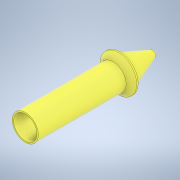
# Autodesk Inventor part: Static Marker Barrel
Saved by Autodesk Inventor 2022.2 (Build 262287010, 287A)
## iProperties
Created: 2022-02-09
Part Number: Static Marker Barrel
Material: ABS Plastic
Document SubType Name: Modeling
Designer: smiku
Density: 1.06 g/cm^3
Appearance: Smooth - Yellow
Author: smiku
Autodesk Inventor part; units mm, degrees
ref_plane "YZ Plane" through (0, 0, 0) normal (1, 0, 0) x (0, 1, 0)
ref_plane "XZ Plane" through (0, 0, 0) normal (0, 1, 0) x (-1, 0, 0)
ref_plane "XY Plane" through (0, 0, 0) normal (0, 0, 1) x (1, 0, 0)
sketch "Sketch1" plane through (0, 0, 0) normal (0, 0, 1) x (1, 0, 0)
  circle A0 centre (0, 0) radius 10
  circle A1 centre (0, 0) radius 11.2
  circle A2 centre (0, 0) radius 15.75
  dimension "d0" = 20
  dimension "d1" = 1.2
  dimension "d12" = 31.5
  dimension "d16" = 22.4
  constraints: 3 centre point, 2 coincident
  measures "d0" diameter of A0
  measures "d1" radial gap between concentric circles of A0 A1
  measures "d12" diameter of A2
  measures "d16" diameter of A1
extrude "Extrusion1" add sketch "Sketch1" against normal blind 31.2 contours A0 | A1 | A2
extrude "Extrusion2" add sketch "Sketch1" along normal blind 80 contours A1
sketch "Sketch2" plane through (0, 0, 0) normal (0, 1, 0) x (-1, 0, 0)
  line L0 (-15.75, -31.2) -> (15.75, -31.2) projected
  line L1 (15.75, 0) -> (-15.75, 0) construction
  line L2 (-15.75, -31.2) -> (15.75, -31.2) projected
  line L3 (15.75, 0) -> (-15.75, 0) projected
  line L4 (15.75, -31.2) -> (15.75, 0) construction
  line L5 (-15.75, -31.2) -> (-15.75, 0) construction
  line L6 (-15.75, 0) -> (-15.75, -31.2) construction
  line L7 (15.75, -1.2) -> (-15.75, -1.2)
  line L8 (15.75, -1.2) -> (15.75, -31.2)
  line L9 (-15.75, -1.2) -> (-15.75, -31.2)
  line L10 (15.75, 0) -> (15.75, -31.2) projected
  arc A0 (15.75, -1.2) -> (12.9532, -3.1146) centre (15.75, -4.2) ccw
  arc A1 (-12.9532, -3.1146) -> (-15.75, -1.2) centre (-15.75, -4.2) ccw
  arc A2 (-2.7968, -29.2854) -> (2.7968, -29.2854) centre (0, -28.2) ccw
  line L11 (2.7968, -29.2854) -> (12.9532, -3.1146)
  line L12 (-12.9532, -3.1146) -> (-2.7968, -29.2854)
  line L13 (0, -31.2) -> (0, -1.2)
  line L14 (-11.2, 0) -> (-11.2, 80) construction
  line L15 (-15.75, 0) -> (-11.2, 4.55)
  line L16 (-11.2, 0) -> (-11.2, 80) projected
  line L17 (-11.2, 4.55) -> (-11.2, 0)
  line L18 (-11.2, 0) -> (-15.75, 0)
  point P0 (0, 0)
  dimension "d7" = 1.2
  dimension "d10" = 3
  dimension "d14" = 45
  constraints: 22 end point, 7 point on circle, 7 tangent, 4 point on line, 3 centre point, 3 collinear, 3 midpoint, 3 vertical, 2 equal radius, 1 coincident, 1 perpendicular
  measures "d7" distance between parallel lines of L1 L7
  measures "d10" radius of A2
  measures "d14" angle of L14 L15
revolve "Revolution1" cut sketch "Sketch2" angle 360 about axis through (0, 0, -31.2) along (0, 0, 1) contours L9 A1 L12 A2 L0
revolve "Revolution2" add sketch "Sketch2" angle 360 about axis through (0, 0, -31.2) along (0, 0, 1) contours L3 L15 L16 | A2 L12 A1 L7 L13
sketch "Sketch3" plane through (0, 0, 0) normal (0, 0, 1) x (1, 0, 0)
  circle A0 centre (0, 0) radius 4.5
  dimension "d17" = 9
  constraints: 1 centre point, 1 coincident
  measures "d17" diameter of A0
extrude "Extrusion4" add sketch "Sketch3" along normal blind 10
body "Solid1"
